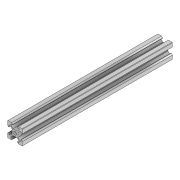
# Autodesk Inventor part: Perfil2020
Saved by Autodesk Inventor 2021 (Build 250183000, 183)
## iProperties
Created: 2021-02-12
Part Number: Perfil2020
Material: Aluminio 6061
Document SubType Name: Modeling
Designer: sddj_
Density: 2.7 g/cm^3
Appearance: Aluminio - Pulido
Author: sddj_
Autodesk Inventor part; units mm, degrees
ref_plane "YZ Plane" through (0, 0, 0) normal (1, 0, 0) x (0, 1, 0)
ref_plane "XZ Plane" through (0, 0, 0) normal (0, 1, 0) x (-1, 0, 0)
ref_plane "XY Plane" through (0, 0, 0) normal (0, 0, 1) x (1, 0, 0)
sketch "Boceto1" plane through (0, 0, 0) normal (0, 0, 1) x (1, 0, 0)
  circle A0 centre (0, 0) radius 2.1
  line L0 (-12, 0) -> (12, 0)
  line L1 (0, 12) -> (0, -12)
  line L2 (0, 3.9) -> (-2.845, 3.9)
  line L3 (-2.845, 3.9) -> (-5.5, 6.555)
  line L4 (-5.5, 6.555) -> (-5.5, 8.195)
  line L5 (-5.5, 8.195) -> (-3.125, 8.195)
  line L6 (-3.125, 8.545) -> (-4.58, 10)
  line L7 (-4.58, 10) -> (-10, 10)
  line L8 (-10, 10) -> (-10, 4.58)
  line L9 (-10, 4.58) -> (-8.545, 3.125)
  line L10 (-8.195, 3.125) -> (-8.195, 5.4887)
  line L11 (-8.195, 5.4887) -> (-6.555, 5.4887)
  line L12 (-6.555, 5.4887) -> (-3.9, 2.8337)
  line L13 (-3.9, 2.8337) -> (-3.9, 0)
  line L14 (0, 3.9) -> (2.845, 3.9)
  line L15 (2.845, 3.9) -> (5.5, 6.555)
  line L16 (5.5, 6.555) -> (5.5, 8.195)
  line L17 (5.5, 8.195) -> (3.125, 8.195)
  line L18 (3.125, 8.545) -> (4.58, 10)
  line L19 (4.58, 10) -> (10, 10)
  line L20 (10, 10) -> (10, 4.58)
  line L21 (10, 4.58) -> (8.545, 3.125)
  line L22 (8.2079, 3.125) -> (8.195, 5.4887)
  line L23 (8.195, 5.4887) -> (6.555, 5.4887)
  line L24 (6.555, 5.4887) -> (3.9, 2.8337)
  line L25 (3.9, 2.8337) -> (3.9, 0)
  line L26 (0, -3.9) -> (-2.845, -3.9)
  line L27 (-2.845, -3.9) -> (-5.5, -6.555)
  line L28 (-5.5, -6.555) -> (-5.5, -8.195)
  line L29 (-5.5, -8.195) -> (-3.125, -8.195)
  line L30 (-3.125, -8.545) -> (-4.58, -10)
  line L31 (-4.58, -10) -> (-10, -10)
  line L32 (-10, -10) -> (-10, -4.58)
  line L33 (-10, -4.58) -> (-8.545, -3.125)
  line L34 (-8.195, -3.125) -> (-8.195, -5.4887)
  line L35 (-8.195, -5.4887) -> (-6.555, -5.4887)
  line L36 (-6.555, -5.4887) -> (-3.9, -2.8337)
  line L37 (-3.9, -2.8337) -> (-3.9, 0)
  line L38 (10, -10) -> (10, -4.58)
  line L39 (4.58, -10) -> (10, -10)
  line L40 (3.125, -8.545) -> (4.58, -10)
  line L41 (5.5, -8.195) -> (3.125, -8.195)
  line L42 (5.5, -6.555) -> (5.5, -8.195)
  line L43 (2.845, -3.9) -> (5.5, -6.555)
  line L44 (0, -3.9) -> (2.845, -3.9)
  line L45 (3.9, -2.8337) -> (3.9, 0)
  line L46 (6.555, -5.4887) -> (3.9, -2.8337)
  line L47 (8.195, -5.4887) -> (6.555, -5.4887)
  line L48 (8.195, -3.125) -> (8.195, -5.4887)
  line L49 (10, -4.58) -> (8.545, -3.125)
  line L50 (-3.125, 8.195) -> (-3.125, 8.545)
  line L51 (-8.195, 3.125) -> (-8.545, 3.125)
  line L52 (3.125, 8.195) -> (3.125, 8.545)
  line L53 (8.195, 3.125) -> (8.545, 3.125)
  line L54 (-3.125, -8.195) -> (-3.125, -8.545)
  line L55 (-8.195, -3.125) -> (-8.545, -3.125)
  line L56 (3.125, -8.195) -> (3.125, -8.545)
  line L57 (8.195, -3.125) -> (8.545, -3.125)
  dimension "d0" = 4.2
  dimension "d1" = 24
  dimension "d2" = 24
  dimension "d3" = 90
  dimension "d5" = 20
  dimension "d11" = 90
  dimension "d18" = 20
  dimension "d29" = 1.5
  dimension "d30" = 1.64
  dimension "d37" = 1.64
  dimension "d42" = 7.8
  dimension "d44" = 11
  dimension "d45" = 9.16
  dimension "d46" = 9.16
  dimension "d47" = 6.25
  dimension "d48" = 6.25
  dimension "d49" = 0.35
  dimension "d51" = 7.8
  dimension "d52" = 0.35
  dimension "d53" = 1.8
  constraints: 116 end point, 41 symmetric about line, 6 perpendicular, 5 parallel, 4 coincident, 4 point on line, 3 midpoint, 2 horizontal, 2 vertical, 1 centre point
  measures "d0" diameter of A0
  measures "d1" distance of L0.start L0.end
  measures "d2" distance of L1.start L1.end
  measures "d3" angle of L18 L6
  measures "d5" distance between parallel lines of L20 L8
  measures "d11" angle of L21 L49
  measures "d18" distance of L32.start L7.end
  measures "d29" distance between parallel lines of L3 L12
  measures "d30" distance of L3.end L4.end
  measures "d37" distance of L10.end L11.end
  measures "d42" distance between parallel lines of L25 L13
  measures "d44" distance between parallel lines of L16 L4
  measures "d45" distance of L19.start L6.end
  measures "d46" distance of L38.end L20.end
  measures "d47" distance between parallel lines of L52 L50
  measures "d48" distance between parallel lines of L55 L51
  measures "d49" distance of L10.start L9.end
  measures "d51" distance between parallel lines of L26 L2
  measures "d52" distance of L5.end L6.start
  measures "d53" distance from line of L20.end L22
extrude "Extrusión1" add sketch "Boceto1" against normal blind 200 contours L0 L45 L46 L47 L48 L57 L49 L38 L39 L40 L56 L41 L42 L43 L44 L1 A0 | A0 L1 L14 L15 L16 L17 L52 L18 L19 L20 L21 L53 L22 L23 L24 L25 L0 | A0 L0 L13 L12 L11 L10 L51 L9 L8 L7 L6 L50 L5 L4 L3 L2 L1 | L1 L26 L27 L28 L29 L54 L30 L31 L32 L33 L55 L34 L35 L36 L37 L0 A0
fillet "Empalme1" radius 0.5 4 edges at (10, 10, -100) (-10, 10, -100) (10, -10, -100) (-10, -10, -100)
